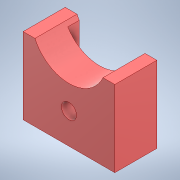
# Autodesk Inventor part: preventWireJumpingSingleSupport
Saved by Autodesk Inventor 2020.2 (Build 242310000, 310)
## iProperties
Created: 2020-02-09
Part Number: preventWireJumpingSingleSupport
Material: PBT Plastic
Document SubType Name: Modeling
Designer: robst
Density: 1.31 g/cm^3
Appearance: Smooth - Red
Author: robst
Autodesk Inventor part; units mm, degrees
ref_plane "YZ Plane" through (0, 0, 0) normal (1, 0, 0) x (0, 1, 0)
ref_plane "XZ Plane" through (0, 0, 0) normal (0, 1, 0) x (-1, 0, 0)
ref_plane "XY Plane" through (0, 0, 0) normal (0, 0, 1) x (1, 0, 0)
sketch "Sketch3" plane through (0, 0, 0) normal (0, 0, 1) x (1, 0, 0)
  line L0 (-12.7, -19.05) -> (12.7, -19.05)
  line L1 (12.7, -19.05) -> (12.7, 19.05)
  line L2 (12.7, 19.05) -> (-12.7, 19.05)
  line L3 (-12.7, 19.05) -> (-12.7, -19.05)
  line L4 (-12.7, -19.05) -> (12.7, 19.05) construction
  line L5 (12.7, -19.05) -> (-12.7, 19.05) construction
  point P0 (0, 0)
  dimension "d0" = 25.4
  dimension "d1" = 38.1
  constraints: 12 end point, 2 midpoint, 2 parallel, 1 horizontal, 1 perpendicular
  measures "d0" distance of L0.start L0.end
  measures "d1" distance of L1.end L0.end
extrude "Extrusion1" add sketch "Sketch3" along normal mid plane 12.7
sketch "Sketch4" plane through (0, 0, 6.35) normal (0, 0, 1) x (1, 0, 0)
  circle A0 centre (0, 0) radius 2.667
  dimension "d4" = 5.334
  constraints: 1 centre point, 1 coincident
  measures "d4" diameter of A0
extrude "Extrusion2" cut sketch "Sketch4" against normal through all
sketch "Sketch5" plane through (-12.7, -19.05, 6.35) normal (-1, 0, 0) x (0, 0, 1)
  line L0 (3.175, 6.35) -> (50.8, 6.35) projected
  line L1 (-12.7, 38.1) -> (-12.7, 0) projected
  line L2 (0, 0) -> (0, 38.1) projected
  line L3 (-12.7, 0) -> (0, 0)
  line L4 (0, 0) -> (0, 6.35)
  line L5 (0, 6.35) -> (-12.7, 6.35)
  line L6 (-12.7, 6.35) -> (-12.7, 0)
  point P0 (-6.35, 19.05)
  point P1 (-12.7, 6.35)
  dimension "d9" = 6.35
  constraints: 8 end point, 2 parallel, 1 horizontal, 1 perpendicular, 1 point on line
  measures "d9" distance between parallel lines of L5 L3
extrude "Extrusion3" cut sketch "Sketch5" against normal through all
sketch "Sketch8" plane through (-12.7, -12.7, -6.35) normal (-1, 0, 0) x (0, 0, 1)
  line L0 (-4.7625, 21.8398) -> (-4.7625, 13.2284) projected
  line L1 (12.7, 0) -> (12.7, 31.75) projected
  line L2 (12.7, 0) -> (-4.7625, 0)
  line L3 (-4.7625, 0) -> (-4.7625, 31.75)
  line L4 (-4.7625, 31.75) -> (12.7, 31.75)
  line L5 (12.7, 31.75) -> (12.7, 0)
  point P0 (6.35, 12.7)
  point P1 (-4.7625, 13.2284)
  constraints: 8 end point, 2 parallel, 1 horizontal, 1 perpendicular
extrude "Extrusion5" add sketch "Sketch8" along normal blind 6.35
mirror "Mirror1" about plane through (0, 0, 0) normal (1, 0, 0) of "Extrusion5"
sketch "Sketch6" plane through (0, 0, 0) normal (0, 0, 1) x (1, 0, 0)
  circle A0 centre (0, 25.4) radius 15.494
  point P0 (0, 0)
  dimension "d10" = 25.4
  dimension "d13" = 30.988
  constraints: 1 centre point, 1 coincident
  measures "d10" distance of point (0, 25.4) point (0, 0)
  measures "d13" diameter of A0
extrude "cutOutForGuide" cut sketch "Sketch6" along normal through all both and the other way through all
sketch "Sketch9" plane through (0, 0, 6.35) normal (0, 0, 1) x (1, 0, 0)
  circle A0 centre (0, 0) radius 3.1242
  dimension "d16" = 6.2484
  constraints: 1 centre point, 1 coincident
  measures "d16" diameter of A0
extrude "Extrusion6" cut sketch "Sketch9" against normal blind 9.525
sketch "Sketch10" plane through (-12.7, -12.7, -11.1125) normal (0, 0, -1) x (-1, 0, 0)
  line L0 (0, 0) -> (6.35, 0) projected
  line L1 (0, 0) -> (0.508, 0)
  line L2 (0.508, 0) -> (0.508, 36.9717)
  line L3 (0.508, 36.9717) -> (0, 36.9717)
  line L4 (0, 36.9717) -> (0, 0)
  point P0 (-12.7, 12.7)
  point P1 (0.508, 0)
  dimension "d19" = 0.508
  constraints: 8 end point, 2 parallel, 1 horizontal, 1 perpendicular
  measures "d19" distance of L3.end L2.end
extrude "Extrusion7" cut sketch "Sketch10" against normal blind 4.7625
mirror "Mirror2" about plane through (0, 0, 0) normal (1, 0, 0) of "Extrusion7"
body "Solid1"
